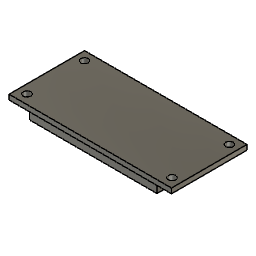
Gehaeuse+Mittelebene+small+feather (Autodesk Fusion 360 archive; units mm, degrees)
design "Adapterplatine Display Groß"
Autodesk Fusion 360 part; units mm, degrees
sketch "Sketch1" plane through (0, 0, 0) normal (0, 0, 1) x (1, 0, 0)
  line L0 (0, 0) -> (65, 0)
  line L1 (65, 0) -> (65, 30.2)
  line L2 (65, 30.2) -> (0, 30.2)
  line L3 (0, 30.2) -> (0, 0)
  line L4 (32.5, 30.2) -> (32.5, 0)
  line L5 (65, 15.1) -> (0, 15.1)
  circle A0 centre (3.5, 26.7) radius 1.5
  circle A1 centre (61.5, 26.7) radius 1.5
  circle A2 centre (3.5, 3.7) radius 1.5
  circle A3 centre (61.5, 3.7) radius 1.5
  line L6 (7, 6.2) -> (58, 6.2)
  line L7 (58, 6.2) -> (58, 1.2)
  line L8 (58, 1.2) -> (7, 1.2)
  line L9 (7, 1.2) -> (7, 6.2)
  dimension "d1" = 65
  dimension "d2" = 30.2
  dimension "d3" = 3
  dimension "d4" = 3.5
  dimension "d5" = 3.5
  dimension "d6" = 3
  dimension "d7" = 3.5
  dimension "d8" = 3.7
  dimension "d11" = 51
  dimension "d12" = 5
  dimension "d14" = 1.2
  constraint horizontal L0
  constraint vertical L1
  constraint horizontal L2
  constraint vertical L3
  constraint coincident L0.start L3.end
  constraint midpoint L2 L4.start
  constraint midpoint L0 L4.end
  constraint midpoint L1 L5.start
  constraint midpoint L3 L5.end
  constraint symmetric L4 A0 A1
  constraint symmetric L4 A2 A3
  constraint horizontal L6
  constraint vertical L7
  constraint horizontal L8
  constraint vertical L9
  constraint symmetric L4 L7 L9
  measures "d1" distance of L0.start L0.end
  measures "d2" distance of L0.start L2.end
  measures "d3" diameter of A0
  measures "d4" distance of L3 A0.centre
  measures "d5" distance of L2 A0.centre
  measures "d6" diameter of A2
  measures "d7" distance of L3 A2.centre
  measures "d8" distance of L0 A2.centre
  measures "d11" distance of L6.start L6.end
  measures "d12" distance of L6.start L8.end
  measures "d14" distance of L0 L8
extrude "Extrude1" add sketch "Sketch1" along normal blind 2
extrude "Extrude2" add sketch "Sketch1" against normal blind 4 contours L4 L6 L8 L9 | L4 L6 L7 L8
